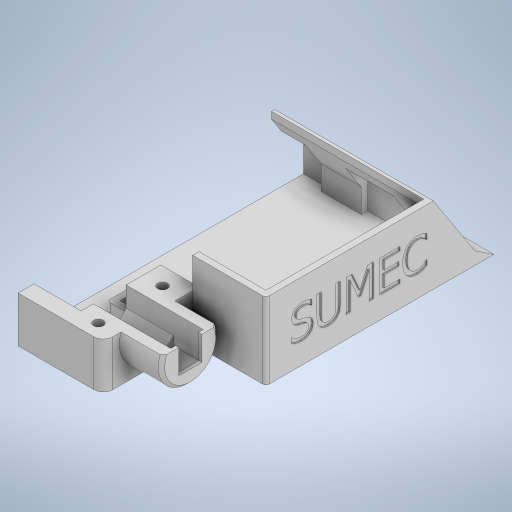
# Autodesk Inventor part: Tělo
Saved by Autodesk Inventor 2024 (Build 280153000, 153)
## iProperties
Created: 2023-04-15
Part Number: Tělo
Material: Všeobecné
Document SubType Name: Modeling
Designer: 42060
Density: 1 g/cm^3
Appearance: Výchozí
Author: 42060
Autodesk Inventor part; units mm, degrees
ref_plane "YZ Plane" through (0, 0, 0) normal (1, 0, 0) x (0, 1, 0)
ref_plane "XZ Plane" through (0, 0, 0) normal (0, 1, 0) x (-1, 0, 0)
ref_plane "XY Plane" through (0, 0, 0) normal (0, 0, 1) x (1, 0, 0)
sketch "Základ" plane through (0, 0, 0) normal (0, 0, 1) x (1, 0, 0)
  line L0 (0, 0) -> (49.75, 0)
  line L1 (49.75, 0) -> (49.75, -71.5)
  line L2 (49.75, -71.5) -> (26.75, -71.5)
  line L3 (26.75, -99.5) -> (0, -99.5)
  line L4 (0, -99.5) -> (0, 0)
  line L5 (0, -20) -> (47.75, -20)
  line L6 (47.75, -20) -> (47.75, -69.5)
  line L7 (47.75, -69.5) -> (14.75, -69.5)
  line L8 (14.75, -69.5) -> (14.75, -94.5)
  line L9 (14.75, -94.5) -> (0, -94.5)
  line L10 (26.75, -71.5) -> (26.75, -80.375)
  line L11 (26.75, -80.375) -> (26.75, -90.625)
  line L12 (26.75, -90.625) -> (26.75, -99.5)
  line L13 (26.75, -90.625) -> (14.75, -90.625)
  line L14 (26.75, -80.375) -> (14.75, -80.375)
  line L15 (26.75, -71.5) -> (26.75, -69.5)
  dimension "d0" = 49.75
  dimension "d1" = 99.5
  dimension "d3" = 2
  dimension "d5" = 28
  dimension "d14" = 10.25
  dimension "d15" = 12
  dimension "d16" = 5
  dimension "d17" = 23
  dimension "d18" = 2
  dimension "d19" = 20
  constraints: 32 end point, 8 perpendicular, 6 point on line, 3 horizontal, 2 collinear, 1 parallel, 1 vertical
  measures "d0" distance of L0.start L0.end
  measures "d1" distance between parallel lines of L3 L0
  measures "d3" distance between parallel lines of L1 L6
  measures "d5" distance of L2.end L3.start
  measures "d14" distance of L10.end L11.end
  measures "d15" distance between parallel lines of L8 L10
  measures "d16" distance between parallel lines of L9 L3
  measures "d17" distance between parallel lines of L1 L12
  measures "d18" distance between parallel lines of L2 L7
  measures "d19" distance between parallel lines of L0 L5
extrude "Podlaha" add sketch "Základ" along normal blind 2 contours L5 L6 L7 L8 L9 L4
extrude "Stěny" add sketch "Základ" along normal blind 24 contours L0 L1 L2 L15 L7 L6 L5 L4
extrude "Zadní stěny" add sketch "Základ" along normal blind 15 contours L9 L8 L13 L12 L3 L4 | L10 L14 L8 L7 L15
extrude "Stěna pod motorem" add sketch "Základ" along normal blind 5.25 contours L11 L13 L8 L14
sketch "Náčrt2" plane through (49.75, -71.5, 0) normal (1, 0, 0) x (0, 0, -1)
  line L0 (-2, 51.5) -> (-24, 51.5) projected
  line L1 (-2, 51.5) -> (-24, 51.5) projected
  line L2 (-24, 0) -> (-24, 71.5) projected
  line L3 (0, 71.5) -> (-24, 71.5) projected
  line L4 (0, 71.5) -> (0, 0) projected
  line L5 (-24, 52.5) -> (-4, 65.5)
  line L6 (-4, 65.5) -> (0, 71.5)
  dimension "d28" = 1
  dimension "d29" = 6
  dimension "d30" = 20
  constraints: 4 end point, 1 point on line
  measures "d28" distance from line of L5.start L0
  measures "d29" vertical distance of L3.start L5.end
  measures "d30" horizontal distance of L5.end L5.start
extrude "Rampa" cut sketch "Náčrt2" against normal through all
sketch "Náčrt3" plane through (0, -20, 2) normal (-1, 0, 0) x (0, 0, 1)
  line L0 (0, 0) -> (22, 0) projected
  line L1 (0, 0) -> (22, 0) projected
  line L2 (19.8687, 0) -> (7.5, 8.0396)
  line L3 (7.5, 8.0396) -> (0, 8.0396)
  line L4 (0, 8.0396) -> (0, 0)
  line L5 (22, 1) -> (2, 14) projected
  point P0 (-2, 20)
  point P1 (19.8687, 0)
  dimension "d34" = 7.5
  dimension "d37" = 2
  constraints: 6 end point, 1 horizontal, 1 parallel, 1 perpendicular, 1 point on line
  measures "d34" distance of L2.end L3.end
  measures "d37" distance between parallel lines of L2 L5
extrude "Přední rampa" cut sketch "Náčrt3" against normal up to surface (47.75 mm away)
sketch "Držák motoru" plane through (14.75, -94.5, 2) normal (-1, 0, 0) x (0, 0, 1)
  line L0 (3.25, 14.125) -> (13, 14.125) projected
  line L1 (3.25, 14.125) -> (3.25, 3.875) projected
  line L2 (3.25, 3.875) -> (13, 3.875) projected
  line L3 (6.13, 14.125) -> (12.37, 14.125)
  line L4 (12.37, 3.875) -> (6.13, 3.875)
  line L5 (3.25, 3.875) -> (13, 3.875) projected
  arc A0 (12.37, 3.875) -> (12.37, 14.125) centre (9.25, 9) ccw
  arc A1 (6.13, 14.125) -> (6.13, 3.875) centre (9.25, 9) ccw
  line L6 (15.25, 14.125) -> (15.25, 3.875) construction
  circle A2 centre (9.25, 9) radius 9
  line L7 (9.25, 18) -> (0, 18)
  line L8 (0, 0) -> (0, 82.5396) projected
  line L9 (0, 0) -> (13, 0) projected
  line L10 (13, -5) -> (13, 3.875) projected
  line L11 (0, 0) -> (13, 0) projected
  line L12 (0, 0) -> (13, 0) projected
  line L13 (12.37, 14.125) -> (12.37, 17.4419)
  line L14 (12.37, 3.875) -> (12.37, 0.5581)
  line L15 (12.37, 0.5581) -> (12.37, 0)
  line L16 (12.37, 17.4419) -> (12.37, 18)
  line L17 (12.37, 18) -> (9.25, 18)
  point P0 (-2, 94.5)
  point P1 (15.25, 9)
  point P2 (15.25, 9)
  point P3 (3.25, 9)
  point P4 (3.25, 9)
  point P5 (6.13, 3.875)
  point P6 (9.25, 0)
  point P7 (16.7333, 14)
  point P8 (16.7333, 4)
  point P9 (12.37, 0)
  dimension "d38" = 6
  dimension "d39" = 6
  dimension "d41" = 3
  dimension "d48" = 12
  constraints: 18 end point, 9 point on circle, 7 point on line, 4 tangent, 3 centre point, 3 coincident, 3 vertical, 2 horizontal alignment, 2 midpoint, 1 horizontal, 1 perpendicular
  measures "d38" radius of A0
  measures "d39" radius of A1
  measures "d41" radial gap between concentric circles of A2 A0
  measures "d48" distance between parallel lines of L1 L6
sketch "Náčrt10" plane through (14.75, -99.5, 0) normal (1, 0, 0) x (0, 0, -1)
  line L0 (-5.25, 8.875) -> (-15, 8.875) construction
  line L1 (-5.25, 8.875) -> (-17.25, 8.875) construction
  line L2 (-17.25, 8.875) -> (-17.25, 19.125) construction
  line L3 (-17.25, 19.125) -> (-5.25, 19.125) construction
  line L4 (-5.25, 19.125) -> (-5.25, 8.875) construction
  line L5 (-14.37, 8.875) -> (-8.13, 8.875)
  arc A0 (-8.13, 8.875) -> (-8.13, 19.125) centre (-11.25, 14) ccw
  line L6 (-14.37, 19.125) -> (-8.13, 19.125)
  arc A1 (-14.37, 5.5581) -> (-14.37, 22.4419) centre (-11.25, 14) ccw
  line L7 (-14.37, 8.875) -> (-14.37, 5.5581)
  line L8 (-14.37, 19.125) -> (-14.37, 22.4419)
  point P0 (0, 99.5)
  point P1 (-11.25, 19.125)
  point P2 (-11.25, 19.125)
  point P3 (-11.25, 8.875)
  point P4 (-11.25, 8.875)
  dimension "d79" = 12
  dimension "d80" = 6
  dimension "d81" = 18
  constraints: 16 end point, 5 point on line, 4 midpoint, 4 point on circle, 3 coincident, 2 centre point, 2 parallel, 2 perpendicular, 2 vertical alignment, 1 collinear, 1 horizontal, 1 horizontal alignment, 1 tangent
  measures "d79" distance between parallel lines of L4 L2
  measures "d80" radius of A0
  measures "d81" diameter of A1
extrude "Držák motoru (kulaté)" add sketch "Náčrt10" along normal blind 15
sketch "Náčrt11" plane through (29.75, -99.5, 0) normal (1, 0, 0) x (0, 0, -1)
  arc A0 (-8.13, 8.875) -> (-8.13, 19.125) centre (-11.25, 14) ccw projected
  circle A1 centre (-11.25, 14) radius 9
  line L0 (-17.25, 8.875) -> (-5.25, 8.875)
  line L1 (-5.25, 8.875) -> (-5.25, 19.125)
  line L2 (-5.25, 19.125) -> (-17.25, 19.125)
  line L3 (-17.25, 19.125) -> (-17.25, 8.875)
  line L4 (-17.25, 8.875) -> (-5.25, 19.125) construction
  line L5 (-5.25, 8.875) -> (-17.25, 19.125) construction
  line L6 (-14.37, 8.875) -> (-14.37, 5.5581) projected
  line L7 (-14.37, 22.4419) -> (-14.37, 19.125) projected
  point P0 (0, 99.5)
  dimension "d84" = 18
  constraints: 12 end point, 2 midpoint, 2 parallel, 1 centre point, 1 coincident, 1 horizontal, 1 horizontal alignment, 1 perpendicular, 1 tangent
  measures "d84" diameter of A1
extrude "Držák motoru (hranaté)" add sketch "Náčrt11" along normal blind 9.25 contours L0 L1 L2 L7 A1 L6
sketch "Náčrt7" plane through (0, 0, 2) normal (0, 0, 1) x (1, 0, 0)
  line L0 (0, -11.9604) -> (47.75, -11.9604) projected
  line L1 (0, -11.9604) -> (47.75, -11.9604) projected
  line L2 (0, 0) -> (0, -99.5) projected
  line L3 (0, -9.9604) -> (7.5, -9.9604)
  line L4 (7.5, -9.9604) -> (7.5, -16.9604)
  line L5 (7.5, -16.9604) -> (0, -16.9604)
  line L6 (0, -16.9604) -> (0, -9.9604)
  line L7 (20.125, -9.9604) -> (35.125, -9.9604)
  line L8 (35.125, -9.9604) -> (35.125, -16.9604)
  line L9 (35.125, -16.9604) -> (20.125, -16.9604)
  line L10 (20.125, -16.9604) -> (20.125, -9.9604)
  point P0 (27.625, -16.9604)
  point P1 (35.125, -11.9604)
  point P2 (20.125, -11.9604)
  point P3 (0, -16.9604)
  point P4 (7.5, -11.9604)
  dimension "d57" = 20.125
  dimension "d58" = 15
  dimension "d59" = 7.5
  dimension "d60" = 7
  dimension "d61" = 2
  constraints: 16 end point, 4 parallel, 3 point on line, 2 horizontal, 2 perpendicular, 1 midpoint
  measures "d57" horizontal distance of point (27.625, -16.96) L1.end
  measures "d58" distance of L7.start L7.end
  measures "d59" distance of L3.start L3.end
  measures "d60" distance of L7.end L8.end
  measures "d61" distance between parallel lines of L0 L3
extrude "Pření senzory" cut sketch "Náčrt7" along normal blind 15
sketch "Spodní senzory" plane through (0, 0, 2) normal (0, 0, 1) x (1, 0, 0)
  line L0 (7.5, -11.9604) -> (20.125, -11.9604) projected
  line L1 (7.5, -11.9604) -> (7.5, -9.9604) projected
  line L2 (7.5, -9.9604) -> (0, -9.9604) projected
  line L3 (0, -94.5) -> (0, -9.9604) projected
  line L4 (0, -94.5) -> (14.75, -94.5) projected
  line L5 (14.75, -94.5) -> (14.75, -69.5) projected
  line L6 (14.75, -69.5) -> (47.75, -69.5) projected
  line L7 (47.75, -69.5) -> (47.75, -11.9604) projected
  line L8 (35.125, -11.9604) -> (47.75, -11.9604) projected
  line L9 (35.125, -11.9604) -> (35.125, -9.9604) projected
  line L10 (35.125, -9.9604) -> (20.125, -9.9604) projected
  line L11 (20.125, -9.9604) -> (20.125, -11.9604) projected
  line L12 (45.75, -13.9604) -> (41.75, -13.9604)
  line L13 (41.75, -13.9604) -> (41.75, -18.7104)
  line L14 (41.75, -18.7104) -> (45.75, -18.7104)
  line L15 (45.75, -18.7104) -> (45.75, -13.9604)
  line L16 (39.75, -11.9604) -> (39.75, -20.7104)
  line L17 (39.75, -20.7104) -> (47.75, -20.7104)
  line L18 (14.75, -69.5) -> (6.75, -69.5)
  line L19 (6.75, -69.5) -> (6.75, -78.25)
  line L20 (6.75, -78.25) -> (14.75, -78.25)
  line L21 (14.75, -78.25) -> (14.75, -69.5)
  line L22 (12.75, -71.5) -> (8.75, -71.5)
  line L23 (8.75, -71.5) -> (8.75, -76.25)
  line L24 (8.75, -76.25) -> (12.75, -76.25)
  line L25 (12.75, -76.25) -> (12.75, -71.5)
  point P0 (0, 0)
  dimension "d64" = 4
  dimension "d65" = 4.75
  dimension "d66" = 2
  dimension "d67" = 2
  dimension "d70" = 2
  dimension "d71" = 2
  dimension "d100" = 4.75
  dimension "d101" = 4
  dimension "d102" = 2
  dimension "d103" = 2
  dimension "d104" = 2
  dimension "d105" = 2
  constraints: 28 end point, 6 parallel, 4 perpendicular, 3 horizontal, 2 point on line, 1 vertical
  measures "d64" distance of L13.end L14.end
  measures "d65" distance of L14.end L12.start
  measures "d66" distance between parallel lines of L7 L15
  measures "d67" distance between parallel lines of L12 L8
  measures "d70" distance between parallel lines of L16 L13
  measures "d71" distance between parallel lines of L17 L14
  measures "d100" distance of L22.end L23.end
  measures "d101" distance of L22.start L22.end
  measures "d102" distance between parallel lines of L19 L23
  measures "d103" distance between parallel lines of L5 L25
  measures "d104" distance between parallel lines of L20 L24
  measures "d105" distance between parallel lines of L22 L18
extrude "Spodní senzory (díra)" cut sketch "Spodní senzory" against normal through all contours L15 L14 L13 L12 | L25 L24 L23 L22
extrude "Spodní senzory zvýšení" add sketch "Spodní senzory" along normal blind 3 contours L8 L7 L17 L16 | L20 L19 L18 L5
sketch "Náčrt12" plane through (0, 0, 15) normal (0, 0, 1) x (1, 0, 0)
  line L0 (26.75, -80.375) -> (26.75, -71.5) projected
  line L1 (26.75, -69.5) -> (26.75, -71.5) projected
  line L2 (26.75, -69.5) -> (14.75, -69.5) projected
  line L3 (14.75, -69.5) -> (14.75, -80.375) projected
  line L4 (14.75, -80.375) -> (26.75, -80.375) projected
  line L5 (26.75, -99.5) -> (26.75, -90.625) projected
  line L6 (26.75, -90.625) -> (14.75, -90.625) projected
  line L7 (14.75, -90.625) -> (14.75, -94.5) projected
  line L8 (14.75, -94.5) -> (0, -94.5) projected
  line L9 (0, -94.5) -> (0, -99.5) projected
  line L10 (0, -99.5) -> (26.75, -99.5) projected
  point P0 (0, 0)
extrude "Vyrovnání držáku motoru" cut sketch "Náčrt12" against normal up to surface (0.63 mm away)
sketch "Náčrt13" plane through (14.75, -80.375, 14.37) normal (0, 0, 1) x (1, 0, 0)
  line L0 (0, 0) -> (0, 10.875) projected
  line L1 (0, 10.875) -> (12, 10.875) projected
  line L2 (0, -14.125) -> (0, -10.25) projected
  line L3 (0, -10.25) -> (24.25, -10.25) projected
  point P0 (-14.75, 80.375)
  point P1 (6, 5.4375)
  point P2 (6, -14.6875)
  dimension "d89" = 6
  dimension "d90" = 5.4375
  dimension "d91" = 6
  dimension "d92" = 4.4375
  measures "d89" distance from line of L0 point (6, 5.438)
  measures "d90" distance from line of L1 point (6, 5.438)
  measures "d91" distance from line of L2 point (6, -14.687)
  measures "d92" distance from line of L3 point (6, -14.687)
hole "Díry pro objímku motoru" at (20.75, -95.0625, 14.37) at (20.75, -74.9375, 14.37) direction (0, 0, -1) diameter 3 depth 6
fillet "Zaoblení1" radius 3 1 edges at (26.75, -99.5, 7.185)
fillet "Zaoblení2" radius 1 4 edges at (49.75, -71.5, 12) (39.75, -20.7104, 3.5) (6.75, -69.5, 3.5) (6.75, -78.25, 3.5)
sketch "Náčrt14" plane through (39, -99.5, 0) normal (1, 0, 0) x (0, 0, -1)
  line L0 (-14.37, 19.125) -> (-5.25, 19.125) projected
  line L1 (-5.25, 19.125) -> (-5.25, 8.875) projected
  line L2 (-5.25, 8.875) -> (-14.37, 8.875) projected
  line L3 (-14.37, 8.875) -> (-14.37, 5.5581) projected
  arc A0 (-14.37, 5.5581) -> (-14.37, 22.4419) centre (-11.25, 14) ccw projected
  line L4 (-14.37, 22.4419) -> (-14.37, 19.125) projected
  line L5 (-14.37, 10.375) -> (-6.75, 10.375)
  line L6 (-6.75, 10.375) -> (-6.75, 17.625)
  line L7 (-6.75, 17.625) -> (-14.37, 17.625)
  line L8 (-14.37, 8.875) -> (-14.37, 10.375)
  line L9 (-14.37, 17.625) -> (-14.37, 19.125)
  point P0 (0, 99.5)
  dimension "d108" = 1.5
  dimension "d109" = 1.5
  dimension "d110" = 1.5
  constraints: 10 end point, 2 perpendicular, 2 point on line, 2 vertical, 2 vertical alignment
  measures "d108" distance between parallel lines of L5 L2
  measures "d109" distance between parallel lines of L1 L6
  measures "d110" distance between parallel lines of L0 L7
extrude "Vysunutí19" add sketch "Náčrt14" along normal blind 1
chamfer "Zkosení1" distance 1 angle 45 1 edges at (40, -85.5, 2.25)
chamfer "Zkosení2" distance 0.25 angle 45 2 edges at (29.75, -88.4394, 6.0193) (29.75, -82.5606, 6.0193)
sketch "Náčrt15" plane through (49.75, -70.5, 0) normal (1, 0, 0) x (0, 0, -1)
  line L0 (-17.0432, 6.4595) -> (-17.0432, 32.0985) construction
  line L1 (-17.0432, 32.0985) -> (-4.204, 32.0985) construction
  line L2 (-4.204, 32.0985) -> (-4.204, 6.4595) construction
  line L3 (-4.204, 6.4595) -> (-17.0432, 6.4595) construction
  spline S0 degree 2 poles (-6.6866, 10.2601) (-6.6866, 9.1742) (-7.1404, 7.6507) (-7.4646, 6.9781) knots 0 0 0 1 2 2 2
  line L4 (-7.4646, 6.9781) -> (-9.1339, 6.9781)
  line L5 (-9.1339, 6.9781) -> (-9.1339, 7.0754)
  spline S1 degree 2 poles (-9.1339, 7.0754) (-8.5181, 7.7318) (-7.8374, 9.393) (-7.8374, 10.1629) knots 0 0 0 1 2 2 2
  spline S2 degree 2 poles (-7.8374, 10.1629) (-7.8374, 11.265) (-8.7531, 12.3914) (-9.5067, 12.3914) knots 0 0 0 1 2 2 2
  spline S3 degree 2 poles (-9.5067, 12.3914) (-10.1064, 12.3914) (-10.8519, 11.7999) (-11.0383, 11.1597) knots 0 0 0 1 2 2 2
  spline S4 degree 2 poles (-11.0383, 11.1597) (-11.168, 10.6977) (-11.3463, 9.9279) (-11.4921, 9.3525) knots 0 0 0 1 2 2 2
  spline S5 degree 2 poles (-11.4921, 9.3525) (-11.6299, 8.8339) (-12.0432, 8.0154) (-12.3754, 7.6994) knots 0 0 0 1 2 2 2
  spline S6 degree 2 poles (-12.3754, 7.6994) (-12.7077, 7.3914) (-13.5991, 7.0511) (-14.1826, 7.0511) knots 0 0 0 1 2 2 2
  spline S7 degree 2 poles (-14.1826, 7.0511) (-15.3981, 7.0511) (-17.0432, 8.9473) (-17.0432, 10.4141) knots 0 0 0 1 2 2 2
  spline S8 degree 2 poles (-17.0432, 10.4141) (-17.0432, 11.2569) (-16.7109, 12.748) (-16.3949, 13.3882) knots 0 0 0 1 2 2 2
  line L6 (-16.3949, 13.3882) -> (-14.8066, 13.3882)
  line L7 (-14.8066, 13.3882) -> (-14.8066, 13.2909)
  spline S9 degree 2 poles (-14.8066, 13.2909) (-15.2442, 12.8128) (-15.8925, 11.3217) (-15.8925, 10.5033) knots 0 0 0 1 2 2 2
  spline S10 degree 2 poles (-15.8925, 10.5033) (-15.8925, 9.5794) (-15.0254, 8.4368) (-14.3203, 8.4368) knots 0 0 0 1 2 2 2
  spline S11 degree 2 poles (-14.3203, 8.4368) (-13.6882, 8.4368) (-12.9346, 9.1094) (-12.7644, 9.7415) knots 0 0 0 1 2 2 2
  spline S12 degree 2 poles (-12.7644, 9.7415) (-12.651, 10.1629) (-12.3592, 11.3866) (-12.2377, 11.7917) knots 0 0 0 1 2 2 2
  spline S13 degree 2 poles (-12.2377, 11.7917) (-11.9216, 12.8209) (-10.6493, 13.7772) (-9.7174, 13.7772) knots 0 0 0 1 2 2 2
  spline S14 degree 2 poles (-9.7174, 13.7772) (-9.1258, 13.7772) (-7.9913, 13.299) (-7.5942, 12.8695) knots 0 0 0 1 2 2 2
  spline S15 degree 2 poles (-7.5942, 12.8695) (-7.1566, 12.3914) (-6.6866, 11.1759) (-6.6866, 10.2601) knots 0 0 0 1 2 2 2
  spline S16 degree 2 poles (-6.6542, 18.6232) (-6.6542, 17.7399) (-7.1161, 16.4271) (-7.578, 15.9652) knots 0 0 0 1 2 2 2
  spline S17 degree 2 poles (-7.578, 15.9652) (-8.0967, 15.4384) (-9.5553, 15.0089) (-10.625, 15.0089) knots 0 0 0 1 2 2 2
  line L8 (-10.625, 15.0089) -> (-16.8649, 15.0089)
  line L9 (-16.8649, 15.0089) -> (-16.8649, 16.3379)
  line L10 (-16.8649, 16.3379) -> (-10.625, 16.3379)
  spline S18 degree 2 poles (-10.625, 16.3379) (-9.9281, 16.3379) (-8.9881, 16.5162) (-8.6072, 16.7674) knots 0 0 0 1 2 2 2
  spline S19 degree 2 poles (-8.6072, 16.7674) (-8.202, 17.0349) (-7.7887, 17.9587) (-7.7887, 18.6232) knots 0 0 0 1 2 2 2
  spline S20 degree 2 poles (-7.7887, 18.6232) (-7.7887, 19.2472) (-8.202, 20.2196) (-8.6072, 20.487) knots 0 0 0 1 2 2 2
  spline S21 degree 2 poles (-8.6072, 20.487) (-8.9881, 20.7383) (-9.92, 20.9165) (-10.5926, 20.9165) knots 0 0 0 1 2 2 2
  line L11 (-10.5926, 20.9165) -> (-16.8649, 20.9165)
  line L12 (-16.8649, 20.9165) -> (-16.8649, 22.2456)
  line L13 (-16.8649, 22.2456) -> (-10.625, 22.2456)
  spline S22 degree 2 poles (-10.625, 22.2456) (-9.5797, 22.2456) (-8.0886, 21.8242) (-7.578, 21.2893) knots 0 0 0 1 2 2 2
  spline S23 degree 2 poles (-7.578, 21.2893) (-7.108, 20.8112) (-6.6542, 19.547) (-6.6542, 18.6232) knots 0 0 0 1 2 2 2
  line L14 (-6.8649, 32.7237) -> (-6.8649, 31.3947)
  line L15 (-6.8649, 31.3947) -> (-15.4792, 31.3947)
  line L16 (-15.4792, 31.3947) -> (-9.6202, 28.7853)
  line L17 (-9.6202, 28.7853) -> (-9.6202, 27.9749)
  line L18 (-9.6202, 27.9749) -> (-15.4792, 25.3898)
  line L19 (-15.4792, 25.3898) -> (-6.8649, 25.3898)
  line L20 (-6.8649, 25.3898) -> (-6.8649, 24.1499)
  line L21 (-6.8649, 24.1499) -> (-16.8649, 24.1499)
  line L22 (-16.8649, 24.1499) -> (-16.8649, 25.9652)
  line L23 (-16.8649, 25.9652) -> (-11.2976, 28.4611)
  line L24 (-11.2976, 28.4611) -> (-16.8649, 30.876)
  line L25 (-16.8649, 30.876) -> (-16.8649, 32.7237)
  line L26 (-16.8649, 32.7237) -> (-6.8649, 32.7237)
  line L27 (-6.8649, 34.7496) -> (-16.8649, 34.7496)
  line L28 (-16.8649, 34.7496) -> (-16.8649, 41.0057)
  line L29 (-16.8649, 41.0057) -> (-15.6818, 41.0057)
  line L30 (-15.6818, 41.0057) -> (-15.6818, 36.0786)
  line L31 (-15.6818, 36.0786) -> (-12.9427, 36.0786)
  line L32 (-12.9427, 36.0786) -> (-12.9427, 40.6734)
  line L33 (-12.9427, 40.6734) -> (-11.7596, 40.6734)
  line L34 (-11.7596, 40.6734) -> (-11.7596, 36.0786)
  line L35 (-11.7596, 36.0786) -> (-8.048, 36.0786)
  line L36 (-8.048, 36.0786) -> (-8.048, 41.0057)
  line L37 (-8.048, 41.0057) -> (-6.8649, 41.0057)
  line L38 (-6.8649, 41.0057) -> (-6.8649, 34.7496)
  spline S24 degree 2 poles (-6.6866, 46.3704) (-6.6866, 45.3979) (-7.343, 43.7529) (-7.9994, 43.1532) knots 0 0 0 1 2 2 2
  spline S25 degree 2 poles (-7.9994, 43.1532) (-8.6477, 42.5535) (-10.5926, 41.8971) (-11.8568, 41.8971) knots 0 0 0 1 2 2 2
  spline S26 degree 2 poles (-11.8568, 41.8971) (-13.1129, 41.8971) (-14.9767, 42.5373) (-15.6656, 43.1451) knots 0 0 0 1 2 2 2
  spline S27 degree 2 poles (-15.6656, 43.1451) (-16.3382, 43.7447) (-17.0432, 45.3817) (-17.0432, 46.3947) knots 0 0 0 1 2 2 2
  spline S28 degree 2 poles (-17.0432, 46.3947) (-17.0432, 46.8971) (-16.8973, 47.7804) (-16.7839, 48.1532) knots 0 0 0 1 2 2 2
  spline S29 degree 2 poles (-16.7839, 48.1532) (-16.6785, 48.4773) (-16.3787, 49.1499) (-16.2004, 49.4822) knots 0 0 0 1 2 2 2
  line L39 (-16.2004, 49.4822) -> (-14.5959, 49.4822)
  line L40 (-14.5959, 49.4822) -> (-14.5959, 49.3768)
  spline S30 degree 2 poles (-14.5959, 49.3768) (-14.7579, 49.1986) (-15.2117, 48.6475) (-15.4305, 48.2504) knots 0 0 0 1 2 2 2
  spline S31 degree 2 poles (-15.4305, 48.2504) (-15.6412, 47.8695) (-15.9087, 46.97) (-15.9087, 46.3866) knots 0 0 0 1 2 2 2
  spline S32 degree 2 poles (-15.9087, 46.3866) (-15.9087, 45.7464) (-15.3819, 44.6037) (-14.8795, 44.1742) knots 0 0 0 1 2 2 2
  spline S33 degree 2 poles (-14.8795, 44.1742) (-14.369, 43.7529) (-12.8211, 43.2828) (-11.8568, 43.2828) knots 0 0 0 1 2 2 2
  spline S34 degree 2 poles (-11.8568, 43.2828) (-10.8276, 43.2828) (-9.3446, 43.7772) (-8.8341, 44.2067) knots 0 0 0 1 2 2 2
  spline S35 degree 2 poles (-8.8341, 44.2067) (-8.3398, 44.6281) (-7.8374, 45.7545) (-7.8374, 46.3866) knots 0 0 0 1 2 2 2
  spline S36 degree 2 poles (-7.8374, 46.3866) (-7.8374, 46.9619) (-8.121, 47.9425) (-8.3317, 48.3234) knots 0 0 0 1 2 2 2
  spline S37 degree 2 poles (-8.3317, 48.3234) (-8.5424, 48.688) (-8.98, 49.231) (-9.1339, 49.3849) knots 0 0 0 1 2 2 2
  line L41 (-9.1339, 49.3849) -> (-9.1339, 49.4822)
  line L42 (-9.1339, 49.4822) -> (-7.5456, 49.4822)
  spline S38 degree 2 poles (-7.5456, 49.4822) (-7.3916, 49.1499) (-7.108, 48.5665) (-6.9784, 48.1532) knots 0 0 0 1 2 2 2
  spline S39 degree 2 poles (-6.9784, 48.1532) (-6.8325, 47.7156) (-6.6866, 46.97) (-6.6866, 46.3704) knots 0 0 0 1 2 2 2
  point P0 (0, 70.5)
  constraints: 2 other
emboss "Reliéf1" sketch "Náčrt15" operation cut depth 0.4 direction (-1, 0, 0)
